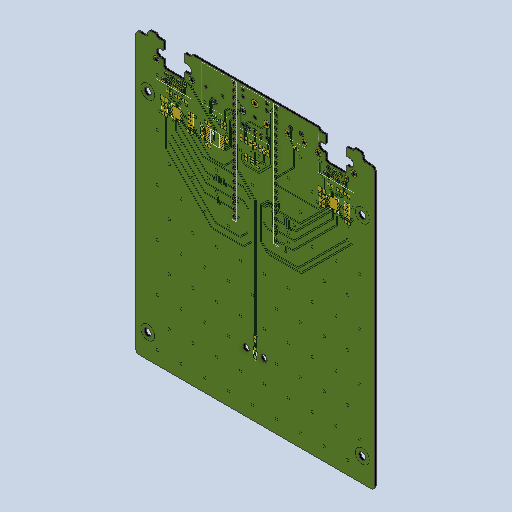
# Autodesk Inventor part: BaseBoard_BOARD
Saved by Autodesk Inventor 2022.2 (Build 262287010, 287A)
## iProperties
Created: 2022-03-22
Part Number: BaseBoard_BOARD
Material: Generic
Document SubType Name: Modeling
Designer: Graeme
Density: 1 g/cm^3
Appearance: BoardColor
Author: Graeme
Autodesk Inventor part; units mm, degrees
ref_plane "YZ Plane" through (0, 0, 0) normal (1, 0, 0) x (0, 1, 0)
ref_plane "XZ Plane" through (0, 0, 0) normal (0, 1, 0) x (-1, 0, 0)
ref_plane "BoardFrontPlane" through (0, 0, 0) normal (0, 0, 1) x (1, 0, 0)
sketch "Sketch1" plane through (0, 0, 0) normal (0, 0, 1) x (1, 0, 0)
  arc A0 (21.06, 5.735) -> (22.33, 4.465) centre (22.33, 5.735) ccw
  line L0 (22.33, 4.465) -> (119.79, 4.465)
  arc A1 (119.79, 4.465) -> (121.06, 5.735) centre (119.79, 5.735) ccw
  line L1 (121.06, 5.735) -> (121.06, 120.425)
  arc A2 (121.06, 120.425) -> (119.79, 121.695) centre (119.79, 120.425) ccw
  line L2 (119.79, 121.695) -> (117.33, 121.695)
  arc A3 (116.06, 122.965) -> (117.33, 121.695) centre (117.33, 122.965) ccw
  line L3 (116.06, 122.965) -> (116.06, 123.195)
  arc A4 (116.06, 123.195) -> (114.79, 124.465) centre (114.79, 123.195) ccw
  line L4 (114.79, 124.465) -> (27.33, 124.465)
  arc A5 (27.33, 124.465) -> (26.06, 123.195) centre (27.33, 123.195) ccw
  line L5 (26.06, 123.195) -> (26.06, 122.965)
  arc A6 (24.79, 121.695) -> (26.06, 122.965) centre (24.79, 122.965) ccw
  line L6 (24.79, 121.695) -> (22.33, 121.695)
  arc A7 (22.33, 121.695) -> (21.06, 120.425) centre (22.33, 120.425) ccw
  line L7 (21.06, 120.425) -> (21.06, 5.735)
  constraints: 16 end point, 16 point on circle, 8 centre point
extrude "BoardOutline" add sketch "Sketch1" along normal blind 0.798
sketch "Sketch8" plane through (0, 0, 0.798) normal (0, 0, 1) x (1, 0, 0)
  point P0 (54.515, 111.615)
hole "J4-1" at (54.515, 111.615, 0.798) direction (0, 0, -1) diameter 0.6 end through all
sketch "Sketch9" plane through (0, 0, 0.798) normal (0, 0, 1) x (1, 0, 0)
  point P0 (53.315, 111.615)
hole "J4-2" at (53.315, 111.615, 0.798) direction (0, 0, -1) diameter 0.6 end through all
sketch "Sketch10" plane through (0, 0, 0.798) normal (0, 0, 1) x (1, 0, 0)
  point P0 (53.315, 112.815)
hole "J4-3" at (53.315, 112.815, 0.798) direction (0, 0, -1) diameter 0.6 end through all
sketch "Sketch11" plane through (0, 0, 0.798) normal (0, 0, 1) x (1, 0, 0)
  point P0 (54.515, 112.815)
hole "J4-4" at (54.515, 112.815, 0.798) direction (0, 0, -1) diameter 0.6 end through all
sketch "Sketch12" plane through (0, 0, 0.798) normal (0, 0, 1) x (1, 0, 0)
  point P0 (57.415, 115.815)
hole "J4-5" at (57.415, 115.815, 0.798) direction (0, 0, -1) diameter 1 end through all
sketch "Sketch13" plane through (0, 0, 0.798) normal (0, 0, 1) x (1, 0, 0)
  point P0 (50.415, 115.815)
hole "J4-6" at (50.415, 115.815, 0.798) direction (0, 0, -1) diameter 1 end through all
sketch "Sketch53" plane through (0, 0, 0.798) normal (0, 0, 1) x (1, 0, 0)
  point P0 (79.95, 74.67)
hole "J2-21" at (79.95, 74.67, 0.798) direction (0, 0, -1) diameter 1.04 end through all
sketch "Sketch54" plane through (0, 0, 0.798) normal (0, 0, 1) x (1, 0, 0)
  point P0 (79.95, 77.21)
hole "J2-22" at (79.95, 77.21, 0.798) direction (0, 0, -1) diameter 1.04 end through all
sketch "Sketch55" plane through (0, 0, 0.798) normal (0, 0, 1) x (1, 0, 0)
  point P0 (79.95, 79.75)
hole "J2-23" at (79.95, 79.75, 0.798) direction (0, 0, -1) diameter 1.04 end through all
sketch "Sketch56" plane through (0, 0, 0.798) normal (0, 0, 1) x (1, 0, 0)
  point P0 (79.95, 82.29)
hole "J2-24" at (79.95, 82.29, 0.798) direction (0, 0, -1) diameter 1.04 end through all
sketch "Sketch57" plane through (0, 0, 0.798) normal (0, 0, 1) x (1, 0, 0)
  point P0 (79.95, 84.83)
hole "J2-25" at (79.95, 84.83, 0.798) direction (0, 0, -1) diameter 1.04 end through all
sketch "Sketch58" plane through (0, 0, 0.798) normal (0, 0, 1) x (1, 0, 0)
  point P0 (79.95, 87.37)
hole "J2-26" at (79.95, 87.37, 0.798) direction (0, 0, -1) diameter 1.04 end through all
sketch "Sketch59" plane through (0, 0, 0.798) normal (0, 0, 1) x (1, 0, 0)
  point P0 (79.95, 89.91)
hole "J2-27" at (79.95, 89.91, 0.798) direction (0, 0, -1) diameter 1.04 end through all
sketch "Sketch60" plane through (0, 0, 0.798) normal (0, 0, 1) x (1, 0, 0)
  point P0 (79.95, 92.45)
hole "J2-28" at (79.95, 92.45, 0.798) direction (0, 0, -1) diameter 1.04 end through all
sketch "Sketch61" plane through (0, 0, 0.798) normal (0, 0, 1) x (1, 0, 0)
  point P0 (79.95, 94.99)
hole "J2-29" at (79.95, 94.99, 0.798) direction (0, 0, -1) diameter 1.04 end through all
sketch "Sketch62" plane through (0, 0, 0.798) normal (0, 0, 1) x (1, 0, 0)
  point P0 (79.95, 97.53)
hole "J2-30" at (79.95, 97.53, 0.798) direction (0, 0, -1) diameter 1.04 end through all
sketch "Sketch63" plane through (0, 0, 0.798) normal (0, 0, 1) x (1, 0, 0)
  point P0 (79.95, 100.07)
hole "J2-31" at (79.95, 100.07, 0.798) direction (0, 0, -1) diameter 1.04 end through all
sketch "Sketch64" plane through (0, 0, 0.798) normal (0, 0, 1) x (1, 0, 0)
  point P0 (79.95, 102.61)
hole "J2-32" at (79.95, 102.61, 0.798) direction (0, 0, -1) diameter 1.04 end through all
sketch "Sketch65" plane through (0, 0, 0.798) normal (0, 0, 1) x (1, 0, 0)
  point P0 (79.95, 105.15)
hole "J2-33" at (79.95, 105.15, 0.798) direction (0, 0, -1) diameter 1.04 end through all
sketch "Sketch66" plane through (0, 0, 0.798) normal (0, 0, 1) x (1, 0, 0)
  point P0 (79.95, 107.69)
hole "J2-34" at (79.95, 107.69, 0.798) direction (0, 0, -1) diameter 1.04 end through all
sketch "Sketch67" plane through (0, 0, 0.798) normal (0, 0, 1) x (1, 0, 0)
  point P0 (79.95, 110.23)
hole "J2-35" at (79.95, 110.23, 0.798) direction (0, 0, -1) diameter 1.04 end through all
sketch "Sketch68" plane through (0, 0, 0.798) normal (0, 0, 1) x (1, 0, 0)
  point P0 (79.95, 112.77)
hole "J2-36" at (79.95, 112.77, 0.798) direction (0, 0, -1) diameter 1.04 end through all
sketch "Sketch69" plane through (0, 0, 0.798) normal (0, 0, 1) x (1, 0, 0)
  point P0 (79.95, 115.31)
hole "J2-37" at (79.95, 115.31, 0.798) direction (0, 0, -1) diameter 1.04 end through all
sketch "Sketch70" plane through (0, 0, 0.798) normal (0, 0, 1) x (1, 0, 0)
  point P0 (79.95, 117.85)
hole "J2-38" at (79.95, 117.85, 0.798) direction (0, 0, -1) diameter 1.04 end through all
sketch "Sketch71" plane through (0, 0, 0.798) normal (0, 0, 1) x (1, 0, 0)
  point P0 (79.95, 120.39)
hole "J2-39" at (79.95, 120.39, 0.798) direction (0, 0, -1) diameter 1.04 end through all
sketch "Sketch72" plane through (0, 0, 0.798) normal (0, 0, 1) x (1, 0, 0)
  point P0 (79.95, 122.93)
hole "J2-40" at (79.95, 122.93, 0.798) direction (0, 0, -1) diameter 1.04 end through all
sketch "Sketch73" plane through (0, 0, 0.798) normal (0, 0, 1) x (1, 0, 0)
  point P0 (62.17, 122.93)
hole "J1-1" at (62.17, 122.93, 0.798) direction (0, 0, -1) diameter 1.04 end through all
sketch "Sketch74" plane through (0, 0, 0.798) normal (0, 0, 1) x (1, 0, 0)
  point P0 (62.17, 120.39)
hole "J1-2" at (62.17, 120.39, 0.798) direction (0, 0, -1) diameter 1.04 end through all
sketch "Sketch75" plane through (0, 0, 0.798) normal (0, 0, 1) x (1, 0, 0)
  point P0 (62.17, 117.85)
hole "J1-3" at (62.17, 117.85, 0.798) direction (0, 0, -1) diameter 1.04 end through all
sketch "Sketch76" plane through (0, 0, 0.798) normal (0, 0, 1) x (1, 0, 0)
  point P0 (62.17, 115.31)
hole "J1-4" at (62.17, 115.31, 0.798) direction (0, 0, -1) diameter 1.04 end through all
sketch "Sketch77" plane through (0, 0, 0.798) normal (0, 0, 1) x (1, 0, 0)
  point P0 (62.17, 112.77)
hole "J1-5" at (62.17, 112.77, 0.798) direction (0, 0, -1) diameter 1.04 end through all
sketch "Sketch78" plane through (0, 0, 0.798) normal (0, 0, 1) x (1, 0, 0)
  point P0 (62.17, 110.23)
hole "J1-6" at (62.17, 110.23, 0.798) direction (0, 0, -1) diameter 1.04 end through all
sketch "Sketch79" plane through (0, 0, 0.798) normal (0, 0, 1) x (1, 0, 0)
  point P0 (62.17, 107.69)
hole "J1-7" at (62.17, 107.69, 0.798) direction (0, 0, -1) diameter 1.04 end through all
sketch "Sketch80" plane through (0, 0, 0.798) normal (0, 0, 1) x (1, 0, 0)
  point P0 (62.17, 105.15)
hole "J1-8" at (62.17, 105.15, 0.798) direction (0, 0, -1) diameter 1.04 end through all
sketch "Sketch81" plane through (0, 0, 0.798) normal (0, 0, 1) x (1, 0, 0)
  point P0 (62.17, 102.61)
hole "J1-9" at (62.17, 102.61, 0.798) direction (0, 0, -1) diameter 1.04 end through all
sketch "Sketch82" plane through (0, 0, 0.798) normal (0, 0, 1) x (1, 0, 0)
  point P0 (62.17, 100.07)
hole "J1-10" at (62.17, 100.07, 0.798) direction (0, 0, -1) diameter 1.04 end through all
sketch "Sketch83" plane through (0, 0, 0.798) normal (0, 0, 1) x (1, 0, 0)
  point P0 (62.17, 97.53)
hole "J1-11" at (62.17, 97.53, 0.798) direction (0, 0, -1) diameter 1.04 end through all
sketch "Sketch84" plane through (0, 0, 0.798) normal (0, 0, 1) x (1, 0, 0)
  point P0 (62.17, 94.99)
hole "J1-12" at (62.17, 94.99, 0.798) direction (0, 0, -1) diameter 1.04 end through all
sketch "Sketch85" plane through (0, 0, 0.798) normal (0, 0, 1) x (1, 0, 0)
  point P0 (62.17, 92.45)
hole "J1-13" at (62.17, 92.45, 0.798) direction (0, 0, -1) diameter 1.04 end through all
sketch "Sketch86" plane through (0, 0, 0.798) normal (0, 0, 1) x (1, 0, 0)
  point P0 (62.17, 89.91)
hole "J1-14" at (62.17, 89.91, 0.798) direction (0, 0, -1) diameter 1.04 end through all
sketch "Sketch87" plane through (0, 0, 0.798) normal (0, 0, 1) x (1, 0, 0)
  point P0 (62.17, 87.37)
hole "J1-15" at (62.17, 87.37, 0.798) direction (0, 0, -1) diameter 1.04 end through all
sketch "Sketch88" plane through (0, 0, 0.798) normal (0, 0, 1) x (1, 0, 0)
  point P0 (62.17, 84.83)
hole "J1-16" at (62.17, 84.83, 0.798) direction (0, 0, -1) diameter 1.04 end through all
sketch "Sketch89" plane through (0, 0, 0.798) normal (0, 0, 1) x (1, 0, 0)
  point P0 (62.17, 82.29)
hole "J1-17" at (62.17, 82.29, 0.798) direction (0, 0, -1) diameter 1.04 end through all
sketch "Sketch90" plane through (0, 0, 0.798) normal (0, 0, 1) x (1, 0, 0)
  point P0 (62.17, 79.75)
hole "J1-18" at (62.17, 79.75, 0.798) direction (0, 0, -1) diameter 1.04 end through all
sketch "Sketch91" plane through (0, 0, 0.798) normal (0, 0, 1) x (1, 0, 0)
  point P0 (62.17, 77.21)
hole "J1-19" at (62.17, 77.21, 0.798) direction (0, 0, -1) diameter 1.04 end through all
sketch "Sketch92" plane through (0, 0, 0.798) normal (0, 0, 1) x (1, 0, 0)
  point P0 (62.17, 74.67)
hole "J1-20" at (62.17, 74.67, 0.798) direction (0, 0, -1) diameter 1.04 end through all
sketch "Sketch139" plane through (0, 0, 0.798) normal (0, 0, 1) x (1, 0, 0)
  line L0 (29.435, 124.645) -> (29.435, 126.558)
  line L1 (29.435, 126.558) -> (44.685, 126.558)
  line L2 (44.685, 126.558) -> (44.685, 124.645)
  arc A0 (43.505, 123.465) -> (44.685, 124.645) centre (43.505, 124.645) ccw
  line L3 (43.505, 123.465) -> (41.56, 123.465)
  line L4 (41.56, 123.465) -> (41.56, 120.056)
  line L5 (41.56, 120.056) -> (42.775, 120.056)
  arc A1 (44.405, 118.426) -> (42.775, 120.056) centre (42.775, 118.426) ccw
  arc A2 (42.775, 116.796) -> (44.405, 118.426) centre (42.775, 118.426) ccw
  line L6 (42.775, 116.796) -> (41.56, 116.796)
  line L7 (41.56, 116.796) -> (41.56, 114.845)
  arc A3 (40.38, 113.665) -> (41.56, 114.845) centre (40.38, 114.845) ccw
  line L8 (40.38, 113.665) -> (33.74, 113.665)
  arc A4 (32.56, 114.845) -> (33.74, 113.665) centre (33.74, 114.845) ccw
  line L9 (32.56, 114.845) -> (32.56, 116.796)
  line L10 (32.56, 116.796) -> (31.345, 116.796)
  arc A5 (29.715, 118.426) -> (31.345, 116.796) centre (31.345, 118.426) ccw
  arc A6 (31.345, 120.056) -> (29.715, 118.426) centre (31.345, 118.426) ccw
  line L11 (31.345, 120.056) -> (32.56, 120.056)
  line L12 (32.56, 120.056) -> (32.56, 123.465)
  line L13 (32.56, 123.465) -> (30.615, 123.465)
  arc A7 (29.435, 124.645) -> (30.615, 123.465) centre (30.615, 124.645) ccw
  constraints: 28 end point, 16 point on circle, 8 centre point
extrude "Cutout 1" cut sketch "Sketch139" against normal through all
sketch "Sketch152" plane through (0, 0, 0.798) normal (0, 0, 1) x (1, 0, 0)
  line L0 (97.435, 124.645) -> (97.435, 126.558)
  line L1 (97.435, 126.558) -> (112.685, 126.558)
  line L2 (112.685, 126.558) -> (112.685, 124.645)
  arc A0 (111.505, 123.465) -> (112.685, 124.645) centre (111.505, 124.645) ccw
  line L3 (111.505, 123.465) -> (109.56, 123.465)
  line L4 (109.56, 123.465) -> (109.56, 120.056)
  line L5 (109.56, 120.056) -> (110.775, 120.056)
  arc A1 (112.405, 118.426) -> (110.775, 120.056) centre (110.775, 118.426) ccw
  arc A2 (110.775, 116.796) -> (112.405, 118.426) centre (110.775, 118.426) ccw
  line L6 (110.775, 116.796) -> (109.56, 116.796)
  line L7 (109.56, 116.796) -> (109.56, 114.845)
  arc A3 (108.38, 113.665) -> (109.56, 114.845) centre (108.38, 114.845) ccw
  line L8 (108.38, 113.665) -> (101.74, 113.665)
  arc A4 (100.56, 114.845) -> (101.74, 113.665) centre (101.74, 114.845) ccw
  line L9 (100.56, 114.845) -> (100.56, 116.796)
  line L10 (100.56, 116.796) -> (99.345, 116.796)
  arc A5 (97.715, 118.426) -> (99.345, 116.796) centre (99.345, 118.426) ccw
  arc A6 (99.345, 120.056) -> (97.715, 118.426) centre (99.345, 118.426) ccw
  line L11 (99.345, 120.056) -> (100.56, 120.056)
  line L12 (100.56, 120.056) -> (100.56, 123.465)
  line L13 (100.56, 123.465) -> (98.615, 123.465)
  arc A7 (97.435, 124.645) -> (98.615, 123.465) centre (98.615, 124.645) ccw
  constraints: 28 end point, 16 point on circle, 8 centre point
extrude "Cutout 2" cut sketch "Sketch152" against normal through all
sketch "img_Top" plane through (0, 0, 0.798) normal (0, 0, 1) x (1, 0, 0)
  line L0 (21.06, 124.465) -> (121.0685, 124.465) construction
  line L1 (121.0685, 124.465) -> (121.0685, 4.465) construction
  line L2 (121.0685, 4.465) -> (21.06, 4.465) construction
  line L3 (21.06, 4.465) -> (21.06, 124.465) construction
  constraints: 2 other
decal "Decal_Top"
sketch "img_Bottom" plane through (0, 0, -0.798) normal (0, 0, -1) x (1, 0, 0)
  line L0 (21.06, -4.465) -> (121.0685, -4.465) construction
  line L1 (121.0685, -4.465) -> (121.0685, -124.465) construction
  line L2 (121.0685, -124.465) -> (21.06, -124.465) construction
  line L3 (21.06, -124.465) -> (21.06, -4.465) construction
  constraints: 2 other
decal "Decal_Bottom"
sketch "Sketch155" plane through (0, 0, 0.798) normal (0, 0, 1) x (1, 0, 0)
  point P0 (65.98, 122.465)
hole "J3-MH7" at (65.98, 122.465, 0.798) direction (0, 0, -1) diameter 1.2 end through all
sketch "Sketch156" plane through (0, 0, 0.798) normal (0, 0, 1) x (1, 0, 0)
  point P0 (65.98, 119.965)
hole "J3-MH5" at (65.98, 119.965, 0.798) direction (0, 0, -1) diameter 1.2 end through all
sketch "Sketch157" plane through (0, 0, 0.798) normal (0, 0, 1) x (1, 0, 0)
  point P0 (75.98, 122.465)
hole "J3-MH6" at (75.98, 122.465, 0.798) direction (0, 0, -1) diameter 1.2 end through all
sketch "Sketch158" plane through (0, 0, 0.798) normal (0, 0, 1) x (1, 0, 0)
  point P0 (75.98, 119.965)
hole "J3-MH4" at (75.98, 119.965, 0.798) direction (0, 0, -1) diameter 1.2 end through all
sketch "Sketch159" plane through (0, 0, 0.798) normal (0, 0, 1) x (1, 0, 0)
  point P0 (70.98, 114.965)
hole "J3-MH3" at (70.98, 114.965, 0.798) direction (0, 0, -1) diameter 1.2 end through all
sketch "Sketch160" plane through (0, 0, 0.798) normal (0, 0, 1) x (1, 0, 0)
  point P0 (65.98, 109.965)
hole "J3-MH2" at (65.98, 109.965, 0.798) direction (0, 0, -1) diameter 1.2 end through all
sketch "Sketch161" plane through (0, 0, 0.798) normal (0, 0, 1) x (1, 0, 0)
  point P0 (75.98, 109.965)
hole "J3-MH1" at (75.98, 109.965, 0.798) direction (0, 0, -1) diameter 1.2 end through all
sketch "Sketch162" plane through (0, 0, 0.798) normal (0, 0, 1) x (1, 0, 0)
  point P0 (70.98, 119.965)
hole "J3-1" at (70.98, 119.965, 0.798) direction (0, 0, -1) diameter 1.4 end through all
sketch "Sketch163" plane through (0, 0, 0.798) normal (0, 0, 1) x (1, 0, 0)
  point P0 (73.48, 109.965)
hole "J3-4" at (73.48, 109.965, 0.798) direction (0, 0, -1) diameter 1 end through all
sketch "Sketch164" plane through (0, 0, 0.798) normal (0, 0, 1) x (1, 0, 0)
  point P0 (70.98, 109.965)
hole "J3-5" at (70.98, 109.965, 0.798) direction (0, 0, -1) diameter 1 end through all
sketch "Sketch165" plane through (0, 0, 0.798) normal (0, 0, 1) x (1, 0, 0)
  point P0 (68.48, 109.965)
hole "J3-6" at (68.48, 109.965, 0.798) direction (0, 0, -1) diameter 1 end through all
sketch "Sketch166" plane through (0, 0, 0.798) normal (0, 0, 1) x (1, 0, 0)
  point P0 (65.98, 114.965)
hole "J3-2" at (65.98, 114.965, 0.798) direction (0, 0, -1) diameter 1.4 end through all
sketch "Sketch167" plane through (0, 0, 0.798) normal (0, 0, 1) x (1, 0, 0)
  point P0 (75.98, 114.965)
hole "J3-3" at (75.98, 114.965, 0.798) direction (0, 0, -1) diameter 1.4 end through all
sketch "Sketch168" plane through (0, 0, 0.798) normal (0, 0, 1) x (1, 0, 0)
  point P0 (42.775, 118.426)
hole "J6-MH4" at (42.775, 118.426, 0.798) direction (0, 0, -1) diameter 3.26 end through all
sketch "Sketch169" plane through (0, 0, 0.798) normal (0, 0, 1) x (1, 0, 0)
  point P0 (31.345, 118.426)
hole "J6-MH3" at (31.345, 118.426, 0.798) direction (0, 0, -1) diameter 3.26 end through all
sketch "Sketch170" plane through (0, 0, 0.798) normal (0, 0, 1) x (1, 0, 0)
  point P0 (29.62, 115.376)
hole "J6-MH2" at (29.62, 115.376, 0.798) direction (0, 0, -1) diameter 1.5 end through all
sketch "Sketch171" plane through (0, 0, 0.798) normal (0, 0, 1) x (1, 0, 0)
  point P0 (44.5, 115.376)
hole "J6-MH1" at (44.5, 115.376, 0.798) direction (0, 0, -1) diameter 1.5 end through all
sketch "Sketch172" plane through (0, 0, 0.798) normal (0, 0, 1) x (1, 0, 0)
  point P0 (32.615, 109.536)
hole "J6-8" at (32.615, 109.536, 0.798) direction (0, 0, -1) diameter 0.89 end through all
sketch "Sketch173" plane through (0, 0, 0.798) normal (0, 0, 1) x (1, 0, 0)
  point P0 (33.885, 112.076)
hole "J6-7" at (33.885, 112.076, 0.798) direction (0, 0, -1) diameter 0.89 end through all
sketch "Sketch174" plane through (0, 0, 0.798) normal (0, 0, 1) x (1, 0, 0)
  point P0 (35.155, 109.536)
hole "J6-6" at (35.155, 109.536, 0.798) direction (0, 0, -1) diameter 0.89 end through all
sketch "Sketch175" plane through (0, 0, 0.798) normal (0, 0, 1) x (1, 0, 0)
  point P0 (36.425, 112.076)
hole "J6-5" at (36.425, 112.076, 0.798) direction (0, 0, -1) diameter 0.89 end through all
sketch "Sketch176" plane through (0, 0, 0.798) normal (0, 0, 1) x (1, 0, 0)
  point P0 (37.695, 109.536)
hole "J6-4" at (37.695, 109.536, 0.798) direction (0, 0, -1) diameter 0.89 end through all
sketch "Sketch177" plane through (0, 0, 0.798) normal (0, 0, 1) x (1, 0, 0)
  point P0 (38.965, 112.076)
hole "J6-3" at (38.965, 112.076, 0.798) direction (0, 0, -1) diameter 0.89 end through all
sketch "Sketch178" plane through (0, 0, 0.798) normal (0, 0, 1) x (1, 0, 0)
  point P0 (40.235, 109.536)
hole "J6-2" at (40.235, 109.536, 0.798) direction (0, 0, -1) diameter 0.89 end through all
sketch "Sketch179" plane through (0, 0, 0.798) normal (0, 0, 1) x (1, 0, 0)
  point P0 (41.505, 112.076)
hole "J6-1" at (41.505, 112.076, 0.798) direction (0, 0, -1) diameter 0.89 end through all
sketch "Sketch180" plane through (0, 0, 0.798) normal (0, 0, 1) x (1, 0, 0)
  point P0 (110.775, 118.426)
hole "J5-MH4" at (110.775, 118.426, 0.798) direction (0, 0, -1) diameter 3.26 end through all
sketch "Sketch181" plane through (0, 0, 0.798) normal (0, 0, 1) x (1, 0, 0)
  point P0 (99.345, 118.426)
hole "J5-MH3" at (99.345, 118.426, 0.798) direction (0, 0, -1) diameter 3.26 end through all
sketch "Sketch182" plane through (0, 0, 0.798) normal (0, 0, 1) x (1, 0, 0)
  point P0 (97.62, 115.376)
hole "J5-MH2" at (97.62, 115.376, 0.798) direction (0, 0, -1) diameter 1.5 end through all
sketch "Sketch183" plane through (0, 0, 0.798) normal (0, 0, 1) x (1, 0, 0)
  point P0 (112.5, 115.376)
hole "J5-MH1" at (112.5, 115.376, 0.798) direction (0, 0, -1) diameter 1.5 end through all
sketch "Sketch184" plane through (0, 0, 0.798) normal (0, 0, 1) x (1, 0, 0)
  point P0 (100.615, 109.536)
hole "J5-8" at (100.615, 109.536, 0.798) direction (0, 0, -1) diameter 0.89 end through all
sketch "Sketch185" plane through (0, 0, 0.798) normal (0, 0, 1) x (1, 0, 0)
  point P0 (101.885, 112.076)
hole "J5-7" at (101.885, 112.076, 0.798) direction (0, 0, -1) diameter 0.89 end through all
sketch "Sketch186" plane through (0, 0, 0.798) normal (0, 0, 1) x (1, 0, 0)
  point P0 (103.155, 109.536)
hole "J5-6" at (103.155, 109.536, 0.798) direction (0, 0, -1) diameter 0.89 end through all
sketch "Sketch187" plane through (0, 0, 0.798) normal (0, 0, 1) x (1, 0, 0)
  point P0 (104.425, 112.076)
hole "J5-5" at (104.425, 112.076, 0.798) direction (0, 0, -1) diameter 0.89 end through all
sketch "Sketch188" plane through (0, 0, 0.798) normal (0, 0, 1) x (1, 0, 0)
  point P0 (105.695, 109.536)
hole "J5-4" at (105.695, 109.536, 0.798) direction (0, 0, -1) diameter 0.89 end through all
sketch "Sketch189" plane through (0, 0, 0.798) normal (0, 0, 1) x (1, 0, 0)
  point P0 (106.965, 112.076)
hole "J5-3" at (106.965, 112.076, 0.798) direction (0, 0, -1) diameter 0.89 end through all
sketch "Sketch190" plane through (0, 0, 0.798) normal (0, 0, 1) x (1, 0, 0)
  point P0 (108.235, 109.536)
hole "J5-2" at (108.235, 109.536, 0.798) direction (0, 0, -1) diameter 0.89 end through all
sketch "Sketch191" plane through (0, 0, 0.798) normal (0, 0, 1) x (1, 0, 0)
  point P0 (109.505, 112.076)
hole "J5-1" at (109.505, 112.076, 0.798) direction (0, 0, -1) diameter 0.89 end through all
sketch "Sketch192" plane through (0, 0, 0.798) normal (0, 0, 1) x (1, 0, 0)
  point P0 (26.06, 14.465)
hole "Free-1_FEOXJPHT" at (26.06, 14.465, 0.798) direction (0, 0, -1) diameter 3 end through all
sketch "Sketch193" plane through (0, 0, 0.798) normal (0, 0, 1) x (1, 0, 0)
  point P0 (116.06, 14.465)
hole "Free-1_SDAHNFJX" at (116.06, 14.465, 0.798) direction (0, 0, -1) diameter 3 end through all
sketch "Sketch194" plane through (0, 0, 0.798) normal (0, 0, 1) x (1, 0, 0)
  point P0 (116.06, 101.965)
hole "Free-1_CCSYNVNB" at (116.06, 101.965, 0.798) direction (0, 0, -1) diameter 3 end through all
sketch "Sketch195" plane through (0, 0, 0.798) normal (0, 0, 1) x (1, 0, 0)
  point P0 (26.06, 101.965)
hole "Free-1_NPNJQHMH" at (26.06, 101.965, 0.798) direction (0, 0, -1) diameter 3 end through all
sketch "Sketch196" plane through (0, 0, 0.798) normal (0, 0, 1) x (1, 0, 0)
  point P0 (74.81, 29.465)
hole "Free-MH3" at (74.81, 29.465, 0.798) direction (0, 0, -1) diameter 2.5 end through all
sketch "Sketch197" plane through (0, 0, 0.798) normal (0, 0, 1) x (1, 0, 0)
  point P0 (67.31, 29.465)
hole "Free-MH2" at (67.31, 29.465, 0.798) direction (0, 0, -1) diameter 2.5 end through all
sketch "Sketch198" plane through (0, 0, 0.798) normal (0, 0, 1) x (1, 0, 0)
  point P0 (84.745, 116.115)
hole "S1-MH2" at (84.745, 116.115, 0.798) direction (0, 0, -1) diameter 1.3 end through all
sketch "Sketch199" plane through (0, 0, 0.798) normal (0, 0, 1) x (1, 0, 0)
  point P0 (91.745, 116.115)
hole "S1-MH1" at (91.745, 116.115, 0.798) direction (0, 0, -1) diameter 1.3 end through all
sketch "Sketch200" plane through (0, 0, 0.798) normal (0, 0, 1) x (1, 0, 0)
  point P0 (85.995, 118.665)
hole "S1-2" at (85.995, 118.665, 0.798) direction (0, 0, -1) diameter 1 end through all
sketch "Sketch201" plane through (0, 0, 0.798) normal (0, 0, 1) x (1, 0, 0)
  point P0 (90.495, 118.665)
hole "S1-1" at (90.495, 118.665, 0.798) direction (0, 0, -1) diameter 1 end through all
body "Solid1"
